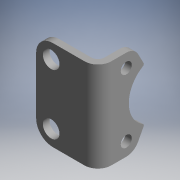
# Autodesk Inventor part: 174370 HNC-40---(F)
Saved by Autodesk Inventor 2017.3 (Build 213256000, 256)
## iProperties
Part Number: 174370 HNC-40---(F)
Material: Generic
Catalog Web Link: www.cadenas.de
Description: HNC-(F)-Foot mounting
Vendor: FESTO
Document SubType Name: Modeling
Designer: partserver
Manufacturer: FESTO
Mass: 193 g
Surface Area: 64.5182 cm^2
Volume: 10.3793 cm^3
Density: 1 g/cm^3
Appearance: PSOLRGB-191-191-191
Category: PARTsolutions
Company: FESTO
Title: 174370 HNC-40
Author: Cadenas PARTsolutions
Comments: Foot mounting
PSOL_IDENT_0: {$CADENAS_DATA\23d-libs\festo\parts\h\hnc\hnc.prj},173 {VTYP=3D},{NB=174370 HNC-40---(F)},{LINA=1743
PSOL_IDENT_1: 70 HNC-40},{NN=HNC-(F)},{DATE=03.09.2015 08:23:22},{GEOMDATE=03.09.2015 08:23:22},{VERSION=},{LINEID=
PSOL_IDENT_2: 20},{WBVAR=},{WBNUMERIC=}  {NB=174370 HNC-40---(F)},{LINA=174370 HNC-40},{KT=DUMMY},{TNR=174370},{TY
PSOL_IDENT_3: P=HNC-40},{KDM=40},{AB=10.000},{AH=36.000},{AW=37.000},{AT=4.000},{AU=28.000},{D2=6.600},{E=54.000},
PSOL_IDENT_4: {LG=18.500},{R1=17.500},{R2=8.000},{TG=38.000},{TG2=19.000},{TR=36.000},{DK=40.000},{D912D=6.000},{D
PSOL_IDENT_5: 912L=18.000},{CNSMASSEXACT=0.193}
NB: 174370 HNC-40---(F)
NN: HNC-(F)
NT: Foot mounting
NBSYN: $TNR. $TYP.---(F)
LINA: 174370 HNC-40
CATALOG: Festo
TNR: 174370
TYP: HNC-40
AB: 10
AH: 36
AW: 37
AT: 4
AU: 28
D2: 6.6
E: 54
LG: 18.5
R1: 17.5
R2: 8
TG: 38
TG2: 19
TR: 36
CNSMASSEXACT: 0.193
SUPPLIER: FESTO
ARTICLENO: 174370 HNC-40---(F)
BOMINFO: 174370 HNC-40
CREATOR: CADENAS GmbH
Autodesk Inventor part; units mm, degrees
sketch "Sketch_1" plane through (0, 0, 0) normal (0, 0, 1) x (1, 0, 0)
  line L0 (0, -1) -> (0, -28)
  arc A0 (0, -28) -> (8, -36) centre (8, -28) ccw
  line L1 (8, -36) -> (37, -36)
  line L2 (37, -36) -> (37, -32)
  line L3 (37, -32) -> (8, -32)
  arc A1 (4, -28) -> (8, -32) centre (8, -28) ccw
  line L4 (4, -28) -> (4, -1)
  line L5 (4, -1) -> (0, -1)
  constraints: 12 end point, 4 point on circle, 2 centre point
extrude "Extrusion1" add sketch "Sketch_1" along normal mid plane 54
sketch "Sketch_2" plane through (0, 0, 0) normal (0, 1, 0) x (-1, 0, 0)
  line L0 (-27, -37) -> (-27, -27)
  arc A0 (-37, -17) -> (-27, -27) centre (-27, -17) ccw
  line L1 (-37, -17) -> (-37, 17)
  arc A1 (-27, 27) -> (-37, 17) centre (-27, 17) ccw
  line L2 (-27, 27) -> (-27, 37)
  line L3 (-27, 37) -> (-47, 37)
  line L4 (-47, 37) -> (-47, -37)
  line L5 (-47, -37) -> (-27, -37)
  constraints: 12 end point, 4 point on circle, 2 centre point
extrude "Extrusion2" cut sketch "Sketch_2" along normal mid plane 74
sketch "Sketch_3" plane through (0, 0, 0) normal (0, 1, 0) x (-1, 0, 0)
  circle A0 centre (-28, -18) radius 5
  constraints: 1 centre point
extrude "Extrusion3" cut sketch "Sketch_3" along normal mid plane 74
sketch "Sketch_4" plane through (0, 0, 0) normal (0, 1, 0) x (-1, 0, 0)
  circle A0 centre (-28, 18) radius 5
  constraints: 1 centre point
extrude "Extrusion4" cut sketch "Sketch_4" along normal mid plane 74
sketch "Sketch_5" plane through (0, 0, 0) normal (1, 0, 0) x (0, 1, 0)
  circle A0 centre (-19, 19) radius 3.3
  constraints: 1 centre point
extrude "Extrusion5" cut sketch "Sketch_5" along normal mid plane 10
sketch "Sketch_6" plane through (0, 0, 0) normal (1, 0, 0) x (0, 1, 0)
  circle A0 centre (-19, -19) radius 3.3
  constraints: 1 centre point
extrude "Extrusion6" cut sketch "Sketch_6" along normal mid plane 10
sketch "Sketch_7" plane through (0, 0, 0) normal (1, 0, 0) x (0, 1, 0)
  line L0 (-41, 32) -> (-41, -32)
  line L1 (-41, -32) -> (0, -32)
  line L2 (0, -32) -> (0, 32)
  line L3 (0, 32) -> (-41, 32)
  line L4 (-19, 27) -> (-36, 27)
  line L5 (-36, 27) -> (-36, -27)
  line L6 (-36, -27) -> (-19, -27)
  arc A0 (-19, -27) -> (-11.9155, -22.7161) centre (-19, -19) ccw
  line L7 (-11.9155, -22.7161) -> (-8.5809, -16.359)
  arc A1 (-8.5809, -16.359) -> (-8.9548, -15.0353) centre (-9.4665, -15.8945) ccw
  arc A2 (-8.9548, 15.0353) -> (-8.9548, -15.0353) centre (0, 0) ccw
  arc A3 (-8.9548, 15.0353) -> (-8.5809, 16.359) centre (-9.4665, 15.8945) ccw
  line L8 (-8.5809, 16.359) -> (-11.9155, 22.7161)
  arc A4 (-11.9155, 22.7161) -> (-19, 27) centre (-19, 19) ccw
  constraints: 18 end point, 10 point on circle, 5 centre point
extrude "Extrusion7" cut sketch "Sketch_7" along normal mid plane 10
ref_plane "HNC_1_XY" through (0, 0, 0) normal (1, 0, 0) x (0, 0, -1)
ref_plane "HNC_1_YZ" through (0, 0, 0) normal (0, 0, -1) x (0, 1, 0)
ref_plane "HNC_1_ZX" through (0, 0, 0) normal (0, 1, 0) x (1, 0, 0)
ref_plane "HNC_2_XY" through (4, -19, 19) normal (1, 0, 0) x (0, 0, -1)
ref_plane "HNC_2_YZ" through (4, -19, 19) normal (0, 0, -1) x (0, 1, 0)
ref_plane "HNC_2_ZX" through (4, -19, 19) normal (0, 1, 0) x (1, 0, 0)
ref_plane "HNC_3_XY" through (4, -19, -19) normal (1, 0, 0) x (0, 0, -1)
ref_plane "HNC_3_YZ" through (4, -19, -19) normal (0, 0, -1) x (0, 1, 0)
ref_plane "HNC_3_ZX" through (4, -19, -19) normal (0, 1, 0) x (1, 0, 0)
ref_plane "P19_XY" through (28, -32, -18) normal (0, 1, 0) x (1, 0, 0)
ref_plane "P19_YZ" through (28, -32, -18) normal (1, 0, 0) x (0, 0, -1)
ref_plane "P19_ZX" through (28, -32, -18) normal (0, 0, -1) x (0, 1, 0)
ref_plane "P20_XY" through (28, -32, 18) normal (0, 1, 0) x (1, 0, 0)
ref_plane "P20_YZ" through (28, -32, 18) normal (1, 0, 0) x (0, 0, -1)
ref_plane "P20_ZX" through (28, -32, 18) normal (0, 0, -1) x (0, 1, 0)
body "Solid1"
